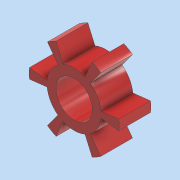
# Autodesk Inventor part: CAO SU KHOP
Saved by Autodesk Inventor 2021 (Build 250183000, 183)
## iProperties
Created: 2022-03-09
Part Number: CAO SU KHOP
Material: Generic
Document SubType Name: Modeling
Designer: 41601100
Density: 1 g/cm^3
Appearance: Default
Author: 41601100
Autodesk Inventor part; units mm, degrees
ref_plane "YZ Plane" through (0, 0, 0) normal (1, 0, 0) x (0, 1, 0)
ref_plane "XZ Plane" through (0, 0, 0) normal (0, 1, 0) x (-1, 0, 0)
ref_plane "XY Plane" through (0, 0, 0) normal (0, 0, 1) x (1, 0, 0)
sketch "Sketch2" plane through (0, 0, 0) normal (0, 0, 1) x (1, 0, 0)
  circle A0 centre (0, 0) radius 14.89
  circle A1 centre (0, 0) radius 9
  circle A2 centre (0, 0) radius 14.89
  line L0 (-3.6007, 8.2483) -> (-5.9571, 13.6464)
  line L1 (5.9571, 13.6464) -> (3.6007, 8.2483)
  circle A3 centre (0, 0) radius 6
  dimension "d10" = 18
  dimension "d12" = 12
  constraints: 4 centre point, 4 end point, 4 point on circle, 1 coincident
  measures "d10" diameter of A1
  measures "d12" diameter of A3
extrude "Extrusion1" add sketch "Sketch2" along normal blind 10.5
extrude "Extrusion2" cut sketch "Sketch2" along normal blind 10.5 contours L1 A1 L0 A0 picked at (-1.0143, 12.8219)
pattern_circular "Circular Pattern1" count 6 over 360 about axis through (0, 0, -10) along (0, 0, 1) of "Extrusion2"
body "Solid1"
